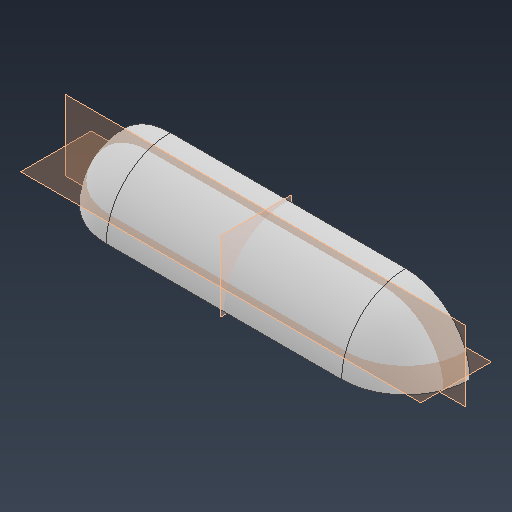
# Autodesk Inventor part: Козырёк_для_камеры
Saved by Autodesk Inventor 2023.2 (Build 272271030, 271C)
## iProperties
Created: 2025-10-07
Part Number: Козырёк_для_камеры
Material: Типовые
Document SubType Name: Modeling
Designer: Олег Коноваленко
Density: 1 g/cm^3
Appearance: По умолчанию
Author: Олег Коноваленко
Autodesk Inventor part; units mm, degrees
sketch "Эскиз3" plane through (0, 0, 0) normal (1, 0, 0) x (0, 1, 0)
  line L0 (-10.6066, -10.6066) -> (-10.6066, 19.3934)
  line L1 (-10.6066, -10.6066) -> (19.3934, -10.6066)
  arc A0 (19.3934, -10.6066) -> (-10.6066, 19.3934) centre (-10.6066, -10.6066) ccw
  line L2 (-10.6066, -10.6066) -> (10.6066, 10.6066) construction
  point P0 (0, 0)
  point P1 (0, 0)
  dimension "d9" = 30
  constraints: 6 end point, 3 point on circle, 2 line through centre, 1 centre point, 1 coincident, 1 horizontal, 1 midpoint, 1 vertical
  measures "d9" distance of L0.start L0.end
extrude "Выдавливание3" add sketch "Эскиз3" along normal mid plane 110
sketch "Эскиз4" plane through (55, 0, 0) normal (1, 0, 0) x (0, 0, -1)
  line L0 (-19.3934, -10.6066) -> (10.6066, -10.6066) projected
  line L1 (10.6066, -10.6066) -> (10.6066, 19.3934) projected
  arc A0 (10.6066, 19.3934) -> (-19.3934, -10.6066) centre (10.6066, -10.6066) ccw projected
  point P0 (0, 0)
revolve "Вращение1" add sketch "Эскиз4" angle 90 about axis through (55, -10.6066, -10.6066) along (0, 1, 0)
mirror "Зеркальное отражение1" about plane through (0, 0, 0) normal (1, 0, 0) of "Вращение1"
shell "Оболочка2" thickness 10 removed faces 2 at (18.3333, -10.6066, -0.6066) at (18.3333, -0.6066, -10.6066)
